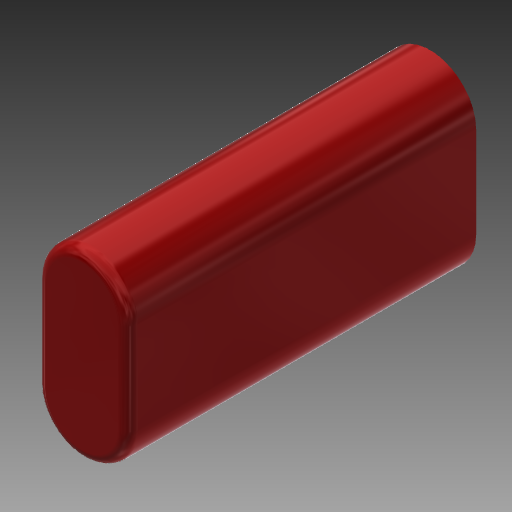
# Autodesk Inventor part: BUSS-SAFTY-TRIP
Saved by Autodesk Inventor 2017.1 (Build 211199000, 199)
## iProperties
Shininess: 64.0
Length Units: 11272
Angle Units: 11279
Time Units: 11290
Mass Units: 11286
Length Display Precision: 3
Angle Display Precision: 2
Compacted: True
Part Number: BUSS-SAFTY-TRIP
Document SubType Name: Modeling
Created: 2003-01-10
Designer: geyerm
Density: 1 g/cm^3
Material: Generic
Appearance: Smooth - Red
Density: 0.0
Volumn: 0.0
Area: 0.0
PropertySet Name: Model Information
Control State: 0
Master: False
Checked Out: False
Author: Autodesk
Autodesk Inventor part; units mm, degrees
ref_plane "YZ Plane" through (0, 0, 0) normal (1, 0, 0) x (0, 1, 0)
ref_plane "XZ Plane" through (0, 0, 0) normal (0, 1, 0) x (-1, 0, 0)
ref_plane "XY Plane" through (0, 0, 0) normal (0, 0, 1) x (1, 0, 0)
sketch "Sketch1" plane through (0, 0, 0) normal (0, 0, 1) x (1, 0, 0)
  arc A0 (-2.159, 14.478) -> (2.159, 14.478) centre (0, 14.478) ccw projected
  line L0 (-2.159, 14.478) -> (-2.159, 17.78) projected
  arc A1 (2.159, 17.78) -> (-2.159, 17.78) centre (0, 17.78) ccw projected
  line L1 (2.159, 17.78) -> (2.159, 14.478) projected
  line L2 (-3.81, -17.78) -> (-3.81, 17.78) projected
  arc A2 (-3.81, -17.78) -> (3.81, -17.78) centre (0, -17.78) ccw projected
  line L3 (3.81, 17.78) -> (3.81, -17.78) projected
  arc A3 (3.81, 17.78) -> (-3.81, 17.78) centre (0, 17.78) ccw projected
  arc A4 (-1.6838, 14.478) -> (1.6838, 14.478) centre (0, 14.478) ccw
  line L4 (-1.6838, 14.478) -> (-1.6838, 17.78)
  arc A5 (1.6838, 17.78) -> (-1.6838, 17.78) centre (0, 17.78) ccw
  line L5 (1.6838, 17.78) -> (1.6838, 14.478)
  constraints: 4 end point, 4 point on circle, 2 centre point, 3 other
extrude "Extrusion1" add sketch "Sketch1" along normal mid plane 12.7 contours L4 A5 L5 A4
fillet "Fillet1" radius 0.381 4 edges at (-1.6838, 16.129, 6.35) (0, 19.4638, 6.35) (1.6838, 16.129, 6.35) (0, 12.7942, 6.35)
body "Solid1"
